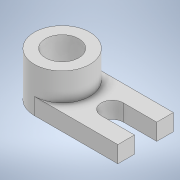
# Autodesk Inventor part: Assignment 3 - Locator
Saved by Autodesk Inventor 2021.1 (Build 251245000, 245)
## iProperties
Created: 2021-05-11
Part Number: Assignment 3 - Locator
Material: Generic
Document SubType Name: Modeling
Designer: as000166
Density: 1 g/cm^3
Appearance: Default
Author: as000166
Autodesk Inventor part; units mm, degrees
ref_plane "YZ Plane" through (0, 0, 0) normal (1, 0, 0) x (0, 1, 0)
ref_plane "XZ Plane" through (0, 0, 0) normal (0, 1, 0) x (-1, 0, 0)
ref_plane "XY Plane" through (0, 0, 0) normal (0, 0, 1) x (1, 0, 0)
sketch "Sketch4" plane through (0, 0, 0) normal (0, 1, 0) x (-1, 0, 0)
  line L0 (-40.1608, 0) -> (34.8392, 0)
  line L1 (34.8392, 0) -> (34.8392, 50)
  line L2 (34.8392, 50) -> (-40.1608, 50)
  line L3 (-40.1608, 50) -> (-40.1608, 0)
  point P0 (0, 0)
  point P1 (0, 0)
  dimension "d3" = 75
  dimension "d4" = 50
  constraints: 8 end point, 2 parallel, 1 horizontal, 1 perpendicular
  measures "d3" distance of L0.start L0.end
  measures "d4" distance of L0.end L1.end
extrude "Extrusion1" add sketch "Sketch4" along normal blind 15
sketch "Sketch5" plane through (0, 0, 0) normal (0, -1, 0) x (1, 0, 0)
  point P0 (0, 0)
sketch "Sketch7" plane through (0, 0, 0) normal (0, -1, 0) x (1, 0, 0)
  line L0 (-34.8392, 0) -> (-34.8392, 50) projected
  circle A0 centre (-35, 25) radius 25.0005
  point P0 (0, 0)
  constraints: 3 other
extrude "Extrusion3" add sketch "Sketch7" against normal blind 40
sketch "Sketch8" plane through (-35, 40, 25) normal (0, 1, 0) x (1, 0, 0)
  circle A0 centre (0, 0) radius 15
  point P0 (35, 25)
  dimension "d11" = 30
  constraints: 1 centre point
  measures "d11" diameter of A0
extrude "Extrusion4" cut sketch "Sketch8" against normal through all
sketch "Sketch9" plane through (0, 15, 0) normal (0, 1, 0) x (1, 0, 0)
  line L0 (40.1608, -50) -> (40.1608, 0) projected
  line L1 (40.1608, 0) -> (-34.8392, 0) projected
  point P0 (0, 0)
  point P1 (10.1608, -25)
  dimension "d14" = 30
  dimension "d15" = 25
  measures "d14" distance from line of L0 point (10.161, -25)
  measures "d15" distance from line of L1 point (10.161, -25)
hole "Hole1" at (10.1608, 15, 25) direction (0, -1, 0) diameter 20 end through all
sketch "Sketch10" plane through (40.1608, 0, 50) normal (1, 0, 0) x (0, 0, -1)
  line L0 (15, 0) -> (15, 15) projected
  line L1 (15, 0) -> (35, 0)
  line L2 (35, 0) -> (35, 15)
  line L3 (35, 15) -> (15, 15)
  line L4 (15, 15) -> (15, 0)
  point P0 (50, 0)
  constraints: 8 end point, 2 parallel, 1 horizontal, 1 perpendicular, 1 point on line
extrude "Extrusion5" cut sketch "Sketch10" against normal up to surface
body "Solid1"
